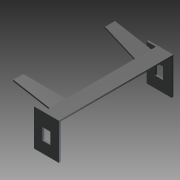
# Autodesk Inventor part: UB216KKW015C-NR
Saved by Autodesk Inventor 2015 SP1 (Build 190203100, 203)
## iProperties
Category: Electrical
Company: Autodesk Inc.
Created: 2014-12-16
Part Number: UB216KKW015C-NR
Catalog Web Link: http://www.nkkswitches.com/
Description: Low Profile Pushbuttons_bodypart_sl-Illuminated Pushbuttons - Series UB2
Vendor: NKK Switches
Document SubType Name: Modeling
Designer: Autodesk Inc.
Manufacturer: NKKSWITCHES
Mass: 0.0186644 g
Surface Area: 1.88722 cm^2
Volume: 0.0186644 cm^3
Density: 1 g/cm^3
Material: Generic
Appearance: PSOLRGB-192-192-192
Title: UB2KKbodypart_sl
Author: Autodesk Inc.
Comments: Illuminated Pushbuttons - Series UB2
Autodesk Inventor part; units mm, degrees
sketch "Sketch_1" plane through (0, 0, 7.9756) normal (0, 0, 1) x (1, 0, 0)
  line L0 (-8.2677, 3.0734) -> (-4.8133, 3.0734)
  line L1 (-4.8133, 3.0734) -> (-4.8133, 8.1534)
  line L2 (-4.8133, 8.1534) -> (-8.2677, 8.1534)
  line L3 (-8.2677, 8.1534) -> (-8.2677, 3.0734)
  line L4 (-7.0993, 6.2484) -> (-7.0993, 4.6228)
  line L5 (-7.0993, 4.6228) -> (-5.9817, 4.6228)
  line L6 (-5.9817, 4.6228) -> (-5.9817, 6.2484)
  line L7 (-5.9817, 6.2484) -> (-7.0993, 6.2484)
  constraints: 16 end point
extrude "Extrusion1" add sketch "Sketch_1" against normal blind 0.254
sketch "Sketch_2" plane through (0, 7.9502, 0) normal (0, 1, 0) x (1, 0, 0)
  line L0 (-7.0993, 7.9756) -> (-7.0993, -7.9756)
  line L1 (-7.0993, -7.9756) -> (-4.8133, -7.9756)
  line L2 (-4.8133, -7.9756) -> (-4.8133, 7.9756)
  line L3 (-4.8133, 7.9756) -> (-7.0993, 7.9756)
  constraints: 8 end point
extrude "Extrusion2" add sketch "Sketch_2" along normal blind 0.2032
sketch "Sketch_3" plane through (0, 0, -7.9756) normal (0, 0, 1) x (1, 0, 0)
  line L0 (-8.2677, 3.0734) -> (-4.8133, 3.0734)
  line L1 (-4.8133, 3.0734) -> (-4.8133, 8.1534)
  line L2 (-4.8133, 8.1534) -> (-8.2677, 8.1534)
  line L3 (-8.2677, 8.1534) -> (-8.2677, 3.0734)
  line L4 (-7.0993, 6.2484) -> (-7.0993, 4.6228)
  line L5 (-7.0993, 4.6228) -> (-5.9817, 4.6228)
  line L6 (-5.9817, 4.6228) -> (-5.9817, 6.2484)
  line L7 (-5.9817, 6.2484) -> (-7.0993, 6.2484)
  constraints: 16 end point
extrude "Extrusion3" add sketch "Sketch_3" along normal blind 0.254
sketch "Sketch_5" plane through (0, 0, 0) normal (0, 0, 1) x (1, 0, 0)
  line L0 (-12.0887, 8.8412) -> (-7.0358, 7.9502)
  line L1 (-7.0358, 7.9502) -> (-7.0005, 8.1503)
  line L2 (-7.0005, 8.1503) -> (-12.0534, 9.0413)
  line L3 (-12.0534, 9.0413) -> (-12.0887, 8.8412)
  constraints: 8 end point
extrude "Extrusion4" add sketch "Sketch_5" along normal mid plane 15.4432
sketch "Sketch_6" plane through (0, 7.9502, 0) normal (0, 1, 0) x (1, 0, 0)
  line L0 (-15.494, -7.7216) -> (-6.985, -7.7216)
  line L1 (-6.985, -7.7216) -> (-6.985, -7.0866)
  line L2 (-6.985, -7.0866) -> (-14.732, -7.0866)
  line L3 (-14.732, -7.0866) -> (-14.732, -6.1666)
  line L4 (-14.732, -6.1666) -> (-6.985, -4.8006)
  line L5 (-6.985, -4.8006) -> (-6.985, 4.8006)
  line L6 (-6.985, 4.8006) -> (-14.732, 6.1666)
  line L7 (-14.732, 6.1666) -> (-14.732, 7.0866)
  line L8 (-14.732, 7.0866) -> (-6.985, 7.0866)
  line L9 (-6.985, 7.0866) -> (-6.985, 7.7216)
  line L10 (-6.985, 7.7216) -> (-15.494, 7.7216)
  line L11 (-15.494, 7.7216) -> (-15.494, -7.7216)
  constraints: 24 end point
extrude "Extrusion5" cut sketch "Sketch_6" along normal blind 2.54
ref_plane "metal_to_body_XY" through (-0.508, 0, 0) normal (1, 0, 0) x (0, 0, -1)
ref_plane "metal_to_body_YZ" through (-0.508, 0, 0) normal (0, 0, -1) x (0, 1, 0)
ref_plane "metal_to_body_ZX" through (-0.508, 0, 0) normal (0, 1, 0) x (1, 0, 0)
body "Solid1"
